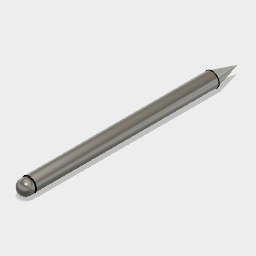
qianbi v1 (Autodesk Fusion 360 design; units mm, degrees)
Autodesk Fusion 360 part; units mm, degrees
cylinder "圆柱体基本要素1" add diameter 8 height 100 placed x (0, 0, -1) y (0, 1, 0) z (1, 0, 0) at (0, 10, 20) makes body 1
sphere "球体基本要素1" add diameter 8 placed x (0, 0, -1) y (0, 1, 0) z (1, 0, 0) at (0, -95, -90) separate body makes body 2
move_body "MoveFace1" bodies 2 to x (1, 0, 0) y (0, 1, 0) z (0, 0, 1) at (-4.2678, 0.1818, 5.1766) on bodies 2
move_face "MoveFace2" to x (1, 0, 0) y (0, 1, 0) z (0, 0, 1) at (0, -97.1967, -1.2623) 1 faces at (66.6667, 9.6017, 16.0199) on bodies 1
move_body "MoveFace3" bodies 2 to x (1, 0, 0) y (0, 1, 0) z (0, 0, 1) at (98.8531, 0, 95.8942) on bodies 2
move_body "MoveFace4" bodies 2 to x (1, 0, 0) y (0, 1, 0) z (0, 0, 1) at (20.7896, 31.3261, -18.2239) on bodies 2
move_body "MoveFace5" bodies 2 to x (1, 0, 0) y (0, 1, 0) z (0, 0, 1) at (8.5994, 0.0217, 49.4172) on bodies 2
move_body "移动1" bodies 1 to x (1, 0, 0) y (0, 1, 0) z (0, 0, 1) at (0, 9.6654, 28.3234)
move_body "移动2" bodies 2 to x (1, 0, 0) y (0, 1, 0) z (0, 0, 1) at (-8.0598, 0, 13.4623)
move_body "对齐1" bodies 1 to x (0, 0, -1) y (0, 1, 0) z (1, 0, 0) at (68.8533, 14.0609, 155.7264)
sketch "草图3" plane through (0, 0, 0) normal (0, 1, 0) x (1, 0, 0)
  line L0 (40, 130) -> (40, 116)
  line L1 (40, 116) -> (44, 116)
  line L2 (44, 116) -> (40, 130)
revolve "旋转1" add sketch "草图3" angle 360 about axis through (40, 0, -130) along (0, 0, 1) separate body makes body 3
move_body "对齐2" bodies 1 to x (1, 0, 0) y (0, 1, 0) z (0, 0, 1) at (-75.9144, 63.4704, -271.7264)
move_face "MoveFace6" to x (1, 0, 0) y (0, 1, 0) z (0, 0, 1) at (-14.3675, 0, 29.6057) 1 faces at (36.0199, -0.3983, -182.6667) on bodies 1
move_body "对齐3" bodies 3 to x (1, 0, 0) y (0, 1, 0) z (0, 0, 1) at (0, 0, 0)
move_body "MoveFace7" bodies 3 to x (1, 0, 0) y (0, 1, 0) z (0, 0, 1) at (-14.155, 0, -99.8779) on bodies 3
move_body "MoveFace8" bodies 2 to x (1, 0, 0) y (0, 1, 0) z (0, 0, 1) at (-90.3426, 63.2398, 0) on bodies 2
move_body "MoveFace9" bodies 2 to x (1, 0, 0) y (0, 1, 0) z (0, 0, 1) at (0.9034, 0, -168.9407) on bodies 2
move_body "MoveFace10" bodies 2 to x (1, 0, 0) y (0, 1, 0) z (0, 0, 1) at (-0.9034, 0, -0.9034) on bodies 2
combine "合并1" operation add target body 2 tool bodies 1
combine "合并2" operation add target body 3 tool bodies 2
